Autodesk Fusion 360 part; units mm, degrees
(part 2 of 2)
sketch "Sketch5" plane through (0, 0, 0) normal (0, -1, 0) x (1, 0, 0)
  line L0 (114.0188, -15.2131) -> (113.0529, -22.5498)
  line L1 (113.0529, -22.5498) -> (82.3181, -18.5035)
  line L2 (82.3181, -18.5035) -> (83.284, -11.1668)
  line L3 (83.284, -11.1668) -> (114.0188, -15.2131)
  line L4 (138.2617, -49.6626) -> (131.6978, -53.0795)
  line L5 (131.6978, -53.0795) -> (117.3836, -25.5822)
  line L6 (117.3836, -25.5822) -> (123.9475, -22.1652)
  line L7 (123.9475, -22.1652) -> (138.2617, -49.6626)
  line L8 (56.4068, -68.2786) -> (77.3501, -91.1342)
  line L9 (77.3501, -91.1342) -> (71.8943, -96.1335)
  line L10 (71.8943, -96.1335) -> (50.951, -73.2779)
  line L11 (50.951, -73.2779) -> (56.4068, -68.2786)
  line L12 (123.9475, -89.2806) -> (117.3836, -85.8637)
  line L13 (117.3836, -85.8637) -> (131.6978, -58.3663)
  line L14 (131.6978, -58.3663) -> (138.2617, -61.7833)
  line L15 (138.2617, -61.7833) -> (123.9475, -89.2806)
  line L16 (83.284, -100.2791) -> (82.3181, -92.9424)
  line L17 (82.3181, -92.9424) -> (113.0529, -88.8961)
  line L18 (113.0529, -88.8961) -> (114.0188, -96.2328)
  line L19 (114.0188, -96.2328) -> (83.284, -100.2791)
  line L20 (71.8943, -15.3123) -> (77.3501, -20.3117)
  line L21 (77.3501, -20.3117) -> (56.4068, -43.1673)
  line L22 (56.4068, -43.1673) -> (50.951, -38.1679)
  line L23 (50.951, -38.1679) -> (71.8943, -15.3123)
  circle A0 centre (93.0518, -55.7229) radius 32
  line L24 (43.0518, -60.3246) -> (33.0518, -60.3246)
  line L25 (33.0518, -60.3246) -> (33.0518, -62.9729)
  arc A1 (33.0518, -62.9729) -> (35.0035, -66.9362) centre (38.0518, -62.9729) ccw
  spline S0 degree 5 poles (35.0035, -66.9362) (35.0877, -67.0016) (35.3696, -67.2106) (35.8903, -67.5453) (36.7154, -67.9795) (37.8844, -68.5138) (39.2185, -69.1644) (40.4642, -69.9451) (41.5622, -70.9096) (42.5171, -72.0738) (43.3656, -73.4352) (44.0003, -74.673) (44.4719, -75.6799) (44.7873, -76.3854) (44.9452, -76.7467) knots 0.055622 0.055622 0.055622 0.055622 0.055622 0.055622 0.1 0.2 0.3 0.4 0.5 0.6 0.7 0.8 0.9 1 1 1 1 1 1
  arc A2 (44.9452, -76.7467) -> (44.6036, -35.4987) centre (93.0518, -55.7229) ccw
  spline S1 degree 5 poles (35.0976, -44.439) (35.1635, -44.39) (35.4284, -44.1998) (35.929, -43.8843) (36.7276, -43.467) (37.8672, -42.9464) (39.2068, -42.2909) (40.468, -41.4976) (41.5888, -40.515) (42.5659, -39.3335) (43.3462, -38.0903) (43.9063, -37.0155) (44.2932, -36.1952) (44.5236, -35.6806) (44.6036, -35.4987) knots 0.065909 0.065909 0.065909 0.065909 0.065909 0.065909 0.1 0.2 0.3 0.4 0.5 0.6 0.7 0.8 0.9 0.95371 0.95371 0.95371 0.95371 0.95371 0.95371
  arc A3 (35.0976, -44.439) -> (33.0518, -48.4729) centre (38.0518, -48.4729) ccw
  line L26 (33.0518, -48.4729) -> (33.0518, -51.3246)
  line L27 (33.0518, -51.3246) -> (43.0518, -51.3246)
  line L28 (43.0518, -51.3246) -> (43.0518, -60.3246)
  circle A4 centre (93.0518, -55.7229) radius 32
  line L29 (56.4068, -43.1673) -> (77.3501, -20.3117)
  line L30 (50.951, -38.1679) -> (56.4068, -43.1673)
  line L31 (71.8943, -15.3123) -> (50.951, -38.1679)
  line L32 (77.3501, -20.3117) -> (71.8943, -15.3123)
  line L33 (113.0529, -88.8961) -> (82.3181, -92.9424)
  line L34 (114.0188, -96.2328) -> (113.0529, -88.8961)
  line L35 (83.284, -100.2791) -> (114.0188, -96.2328)
  line L36 (82.3181, -92.9424) -> (83.284, -100.2791)
  line L37 (131.6978, -58.3663) -> (117.3836, -85.8637)
  line L38 (138.2617, -61.7833) -> (131.6978, -58.3663)
  line L39 (123.9475, -89.2806) -> (138.2617, -61.7833)
  line L40 (117.3836, -85.8637) -> (123.9475, -89.2806)
  line L41 (71.8943, -96.1335) -> (77.3501, -91.1342)
  line L42 (50.951, -73.2779) -> (71.8943, -96.1335)
  line L43 (56.4068, -68.2786) -> (50.951, -73.2779)
  line L44 (77.3501, -91.1342) -> (56.4068, -68.2786)
  line L45 (117.3836, -25.5822) -> (131.6978, -53.0795)
  line L46 (123.9475, -22.1652) -> (117.3836, -25.5822)
  line L47 (138.2617, -49.6626) -> (123.9475, -22.1652)
  line L48 (131.6978, -53.0795) -> (138.2617, -49.6626)
  line L49 (82.3181, -18.5035) -> (113.0529, -22.5498)
  line L50 (83.284, -11.1668) -> (82.3181, -18.5035)
  line L51 (114.0188, -15.2131) -> (83.284, -11.1668)
  line L52 (113.0529, -22.5498) -> (114.0188, -15.2131)
  line L53 (33.0518, -62.9729) -> (33.0518, -60.3246)
  arc A5 (33.0518, -62.9729) -> (35.0035, -66.9362) centre (38.0518, -62.9729) ccw
  spline S2 degree 5 poles (44.9452, -76.7467) (44.7873, -76.3854) (44.4719, -75.6799) (44.0003, -74.673) (43.3656, -73.4352) (42.5171, -72.0738) (41.5622, -70.9096) (40.4642, -69.9451) (39.2185, -69.1644) (37.8844, -68.5138) (36.7154, -67.9795) (35.8903, -67.5453) (35.3696, -67.2106) (35.0877, -67.0016) (35.0035, -66.9362) knots -1 -1 -1 -1 -1 -1 -0.9 -0.8 -0.7 -0.6 -0.5 -0.4 -0.3 -0.2 -0.1 -0.055622 -0.055622 -0.055622 -0.055622 -0.055622 -0.055622
  arc A6 (44.9452, -76.7467) -> (44.6036, -35.4987) centre (93.0518, -55.7229) ccw
  spline S3 degree 5 poles (35.0976, -44.439) (35.1635, -44.39) (35.4284, -44.1998) (35.929, -43.8843) (36.7276, -43.467) (37.8672, -42.9464) (39.2068, -42.2909) (40.468, -41.4976) (41.5888, -40.515) (42.5659, -39.3335) (43.3462, -38.0903) (43.9063, -37.0155) (44.2932, -36.1952) (44.5236, -35.6806) (44.6036, -35.4987) knots 0.065909 0.065909 0.065909 0.065909 0.065909 0.065909 0.1 0.2 0.3 0.4 0.5 0.6 0.7 0.8 0.9 0.95371 0.95371 0.95371 0.95371 0.95371 0.95371
  arc A7 (35.0976, -44.439) -> (33.0518, -48.4729) centre (38.0518, -48.4729) ccw
  line L54 (33.0518, -51.3246) -> (33.0518, -48.4729)
  line L55 (43.0518, -51.3246) -> (33.0518, -51.3246)
  line L56 (43.0518, -60.3246) -> (43.0518, -51.3246)
  line L57 (33.0518, -60.3246) -> (43.0518, -60.3246)
  arc A8 (107.5518, -60.7229) -> (108.5518, -59.7229) centre (107.5518, -59.7229) ccw
  line L58 (105.5518, -60.7229) -> (107.5518, -60.7229)
  arc A9 (105.5518, -60.7229) -> (102.5518, -63.7229) centre (105.5518, -63.7229) ccw
  line L59 (108.5518, -63.7229) -> (102.5518, -63.7229)
  line L60 (108.5518, -66.7229) -> (108.5518, -63.7229)
  line L61 (103.5518, -66.7229) -> (108.5518, -66.7229)
  line L62 (103.5518, -69.7229) -> (103.5518, -66.7229)
  line L63 (108.5518, -69.7229) -> (103.5518, -69.7229)
  line L64 (108.5518, -72.7229) -> (108.5518, -69.7229)
  line L65 (93.5518, -72.7229) -> (108.5518, -72.7229)
  spline S4 degree 2 poles (103.5518, -77.7229) (93.5518, -77.7229) (93.5518, -72.7229) knots -1 -1 -1 0 0 0
  spline S5 degree 2 poles (113.5518, -72.7229) (113.5518, -77.7229) (103.5518, -77.7229) knots 0 0 0 1 1 1
  line L66 (113.5518, -60.7229) -> (113.5518, -72.7229)
  line L67 (113.5518, -44.7229) -> (113.5518, -60.7229)
  arc A10 (113.5518, -44.7229) -> (109.5518, -40.7229) centre (109.5518, -44.7229) ccw
  arc A11 (109.5518, -40.7229) -> (108.5518, -41.7229) centre (109.5518, -41.7229) ccw
  line L68 (108.5518, -59.7229) -> (108.5518, -41.7229)
  arc A12 (99.5518, -49.7229) -> (98.5518, -50.7229) centre (99.5518, -50.7229) ccw
  line L69 (101.5518, -49.7229) -> (99.5518, -49.7229)
  arc A13 (101.5518, -49.7229) -> (104.5518, -46.7229) centre (101.5518, -46.7229) ccw
  line L70 (98.5518, -46.7229) -> (104.5518, -46.7229)
  line L71 (98.5518, -43.7229) -> (98.5518, -46.7229)
  line L72 (103.5518, -43.7229) -> (98.5518, -43.7229)
  line L73 (103.5518, -40.7229) -> (103.5518, -43.7229)
  line L74 (98.5518, -40.7229) -> (103.5518, -40.7229)
  line L75 (98.5518, -37.7229) -> (98.5518, -40.7229)
  line L76 (113.5518, -37.7229) -> (98.5518, -37.7229)
  spline S6 degree 2 poles (103.5518, -32.7229) (113.5518, -32.7229) (113.5518, -37.7229) knots -1 -1 -1 0 0 0
  spline S7 degree 2 poles (93.5518, -37.7229) (93.5518, -32.7229) (103.5518, -32.7229) knots 0 0 0 1 1 1
  line L77 (93.5518, -49.7229) -> (93.5518, -37.7229)
  line L78 (93.5518, -65.7229) -> (93.5518, -49.7229)
  arc A14 (93.5518, -65.7229) -> (97.5518, -69.7229) centre (97.5518, -65.7229) ccw
  arc A15 (97.5518, -69.7229) -> (98.5518, -68.7229) centre (97.5518, -68.7229) ccw
  line L79 (98.5518, -50.7229) -> (98.5518, -68.7229)
  arc A16 (85.0518, -60.7229) -> (86.0518, -59.7229) centre (85.0518, -59.7229) ccw
  line L80 (83.0518, -60.7229) -> (85.0518, -60.7229)
  arc A17 (83.0518, -60.7229) -> (80.0518, -63.7229) centre (83.0518, -63.7229) ccw
  line L81 (86.0518, -63.7229) -> (80.0518, -63.7229)
  line L82 (86.0518, -66.7229) -> (86.0518, -63.7229)
  line L83 (81.0518, -66.7229) -> (86.0518, -66.7229)
  line L84 (81.0518, -69.7229) -> (81.0518, -66.7229)
  line L85 (86.0518, -69.7229) -> (81.0518, -69.7229)
  line L86 (86.0518, -72.7229) -> (86.0518, -69.7229)
  line L87 (71.0518, -72.7229) -> (86.0518, -72.7229)
  spline S8 degree 2 poles (81.0518, -77.7229) (71.0518, -77.7229) (71.0518, -72.7229) knots -1 -1 -1 0 0 0
  spline S9 degree 2 poles (91.0518, -72.7229) (91.0518, -77.7229) (81.0518, -77.7229) knots 0 0 0 1 1 1
  line L88 (91.0518, -60.7229) -> (91.0518, -72.7229)
  line L89 (91.0518, -44.7229) -> (91.0518, -60.7229)
  arc A18 (91.0518, -44.7229) -> (87.0518, -40.7229) centre (87.0518, -44.7229) ccw
  arc A19 (87.0518, -40.7229) -> (86.0518, -41.7229) centre (87.0518, -41.7229) ccw
  line L90 (86.0518, -59.7229) -> (86.0518, -41.7229)
  arc A20 (77.0518, -49.7229) -> (76.0518, -50.7229) centre (77.0518, -50.7229) ccw
  line L91 (79.0518, -49.7229) -> (77.0518, -49.7229)
  arc A21 (79.0518, -49.7229) -> (82.0518, -46.7229) centre (79.0518, -46.7229) ccw
  line L92 (76.0518, -46.7229) -> (82.0518, -46.7229)
  line L93 (76.0518, -43.7229) -> (76.0518, -46.7229)
  line L94 (81.0518, -43.7229) -> (76.0518, -43.7229)
  line L95 (81.0518, -40.7229) -> (81.0518, -43.7229)
  line L96 (76.0518, -40.7229) -> (81.0518, -40.7229)
  line L97 (76.0518, -37.7229) -> (76.0518, -40.7229)
  line L98 (91.0518, -37.7229) -> (76.0518, -37.7229)
  spline S10 degree 2 poles (81.0518, -32.7229) (91.0518, -32.7229) (91.0518, -37.7229) knots -1 -1 -1 0 0 0
  spline S11 degree 2 poles (71.0518, -37.7229) (71.0518, -32.7229) (81.0518, -32.7229) knots 0 0 0 1 1 1
  line L99 (71.0518, -49.7229) -> (71.0518, -37.7229)
  line L100 (71.0518, -65.7229) -> (71.0518, -49.7229)
  arc A22 (71.0518, -65.7229) -> (75.0518, -69.7229) centre (75.0518, -65.7229) ccw
  arc A23 (75.0518, -69.7229) -> (76.0518, -68.7229) centre (75.0518, -68.7229) ccw
  line L101 (76.0518, -50.7229) -> (76.0518, -68.7229)
  circle A24 centre (0, -110) radius 32
  spline S12 degree 5 poles (48.1066, -88.9762) (48.2645, -89.3375) (48.5799, -90.043) (49.0515, -91.0499) (49.6862, -92.2877) (50.5348, -93.6491) (51.4896, -94.8133) (52.5876, -95.7778) (53.8333, -96.5585) (55.1674, -97.2091) (56.3365, -97.7434) (57.1616, -98.1776) (57.6822, -98.5123) (57.9641, -98.7213) (58.0483, -98.7867) knots -1 -1 -1 -1 -1 -1 -0.9 -0.8 -0.7 -0.6 -0.5 -0.4 -0.3 -0.2 -0.1 -0.055622 -0.055622 -0.055622 -0.055622 -0.055622 -0.055622
  arc A25 (48.1066, -88.9762) -> (48.4482, -130.2242) centre (0, -110) ccw
  spline S13 degree 5 poles (57.9542, -121.2839) (57.8883, -121.3329) (57.6234, -121.5231) (57.1228, -121.8387) (56.3243, -122.2559) (55.1846, -122.7765) (53.845, -123.4321) (52.5838, -124.2253) (51.463, -125.2079) (50.4859, -126.3894) (49.7057, -127.6326) (49.1456, -128.7074) (48.7586, -129.5278) (48.5283, -130.0423) (48.4482, -130.2242) knots 0.065909 0.065909 0.065909 0.065909 0.065909 0.065909 0.1 0.2 0.3 0.4 0.5 0.6 0.7 0.8 0.9 0.95371 0.95371 0.95371 0.95371 0.95371 0.95371
  arc A26 (57.9542, -121.2839) -> (60, -117.25) centre (55, -117.25) ccw
  line L102 (60, -102.75) -> (60, -117.25)
  arc A27 (60, -102.75) -> (58.0483, -98.7867) centre (55, -102.75) ccw
  arc A28 (16, -116) -> (17, -115) centre (16, -115) ccw
  line L103 (14, -116) -> (16, -116)
  arc A29 (14, -116) -> (11, -119) centre (14, -119) ccw
  line L104 (17, -119) -> (11, -119)
  line L105 (17, -122) -> (17, -119)
  line L106 (12, -122) -> (17, -122)
  line L107 (12, -125) -> (12, -122)
  line L108 (17, -125) -> (12, -125)
  line L109 (17, -128) -> (17, -125)
  line L110 (2, -128) -> (17, -128)
  spline S14 degree 2 poles (12, -133) (2, -133) (2, -128) knots -1 -1 -1 0 0 0
  spline S15 degree 2 poles (22, -128) (22, -133) (12, -133) knots 0 0 0 1 1 1
  line L111 (22, -116) -> (22, -128)
  line L112 (22, -100) -> (22, -116)
  arc A30 (22, -100) -> (18, -96) centre (18, -100) ccw
  arc A31 (18, -96) -> (17, -97) centre (18, -97) ccw
  line L113 (17, -115) -> (17, -97)
  arc A32 (8, -105) -> (7, -106) centre (8, -106) ccw
  line L114 (10, -105) -> (8, -105)
  arc A33 (10, -105) -> (13, -102) centre (10, -102) ccw
  line L115 (7, -102) -> (13, -102)
  line L116 (7, -99) -> (7, -102)
  line L117 (12, -99) -> (7, -99)
  line L118 (12, -96) -> (12, -99)
  line L119 (7, -96) -> (12, -96)
  line L120 (7, -93) -> (7, -96)
  line L121 (22, -93) -> (7, -93)
  spline S16 degree 2 poles (12, -88) (22, -88) (22, -93) knots -1 -1 -1 0 0 0
  spline S17 degree 2 poles (2, -93) (2, -88) (12, -88) knots 0 0 0 1 1 1
  line L122 (2, -105) -> (2, -93)
  line L123 (2, -121) -> (2, -105)
  arc A34 (2, -121) -> (6, -125) centre (6, -121) ccw
  arc A35 (6, -125) -> (7, -124) centre (6, -124) ccw
  line L124 (7, -106) -> (7, -124)
  arc A36 (-14.5, -105) -> (-15.5, -106) centre (-14.5, -106) ccw
  line L125 (-12.5, -105) -> (-14.5, -105)
  arc A37 (-12.5, -105) -> (-9.5, -102) centre (-12.5, -102) ccw
  line L126 (-15.5, -102) -> (-9.5, -102)
  line L127 (-15.5, -99) -> (-15.5, -102)
  line L128 (-10.5, -99) -> (-15.5, -99)
  line L129 (-10.5, -96) -> (-10.5, -99)
  line L130 (-15.5, -96) -> (-10.5, -96)
  line L131 (-15.5, -93) -> (-15.5, -96)
  line L132 (-0.5, -93) -> (-15.5, -93)
  spline S18 degree 2 poles (-10.5, -88) (-0.5, -88) (-0.5, -93) knots -1 -1 -1 0 0 0
  spline S19 degree 2 poles (-20.5, -93) (-20.5, -88) (-10.5, -88) knots 0 0 0 1 1 1
  line L133 (-20.5, -105) -> (-20.5, -93)
  line L134 (-20.5, -121) -> (-20.5, -105)
  arc A38 (-20.5, -121) -> (-16.5, -125) centre (-16.5, -121) ccw
  arc A39 (-16.5, -125) -> (-15.5, -124) centre (-16.5, -124) ccw
  line L135 (-15.5, -106) -> (-15.5, -124)
  arc A40 (-6.5, -116) -> (-5.5, -115) centre (-6.5, -115) ccw
  line L136 (-8.5, -116) -> (-6.5, -116)
  arc A41 (-8.5, -116) -> (-11.5, -119) centre (-8.5, -119) ccw
  line L137 (-5.5, -119) -> (-11.5, -119)
  line L138 (-5.5, -122) -> (-5.5, -119)
  line L139 (-10.5, -122) -> (-5.5, -122)
  line L140 (-10.5, -125) -> (-10.5, -122)
  line L141 (-5.5, -125) -> (-10.5, -125)
  line L142 (-5.5, -128) -> (-5.5, -125)
  line L143 (-20.5, -128) -> (-5.5, -128)
  spline S20 degree 2 poles (-10.5, -133) (-20.5, -133) (-20.5, -128) knots -1 -1 -1 0 0 0
  spline S21 degree 2 poles (-0.5, -128) (-0.5, -133) (-10.5, -133) knots 0 0 0 1 1 1
  line L144 (-0.5, -116) -> (-0.5, -128)
  line L145 (-0.5, -100) -> (-0.5, -116)
  arc A42 (-0.5, -100) -> (-4.5, -96) centre (-4.5, -100) ccw
  arc A43 (-4.5, -96) -> (-5.5, -97) centre (-4.5, -97) ccw
  line L146 (-5.5, -115) -> (-5.5, -97)
  circle A44 centre (0, 0) radius 32
  line L147 (-1.5, 52.4786) -> (-1.5, 47.5)
  arc A45 (-1.5, 52.4786) -> (-44.6978, 27.5383) centre (0, 0) ccw
  line L148 (-40.3862, 25.049) -> (-44.6978, 27.5383)
  line L149 (-41.8862, 22.451) -> (-40.3862, 25.049)
  line L150 (-46.1978, 24.9402) -> (-41.8862, 22.451)
  arc A46 (-46.1978, 24.9402) -> (-46.1978, -24.9402) centre (0, 0) ccw
  line L151 (-41.8862, -22.451) -> (-46.1978, -24.9402)
  line L152 (-40.3862, -25.049) -> (-41.8862, -22.451)
  line L153 (-44.6978, -27.5383) -> (-40.3862, -25.049)
  arc A47 (-44.6978, -27.5383) -> (-1.5, -52.4786) centre (0, 0) ccw
  line L154 (-1.5, -47.5) -> (-1.5, -52.4786)
  line L155 (1.5, -47.5) -> (-1.5, -47.5)
  line L156 (1.5, -52.4786) -> (1.5, -47.5)
  arc A48 (1.5, -52.4786) -> (44.6978, -27.5383) centre (0, 0) ccw
  line L157 (40.3862, -25.049) -> (44.6978, -27.5383)
  line L158 (41.8862, -22.451) -> (40.3862, -25.049)
  line L159 (46.1978, -24.9402) -> (41.8862, -22.451)
  arc A49 (46.1978, -24.9402) -> (48.1066, -21.0238) centre (0, 0) ccw
  spline S22 degree 5 poles (48.4482, -20.2242) (48.3793, -20.381) (48.3106, -20.5394) (48.2423, -20.6993) (48.1743, -20.8608) (48.1066, -21.0238) knots 0.95371 0.95371 0.95371 0.95371 0.95371 0.95371 1 1 1 1 1 1
  spline S23 degree 5 poles (57.9542, -11.2839) (57.8883, -11.3329) (57.6234, -11.5231) (57.1228, -11.8387) (56.3243, -12.2559) (55.1846, -12.7765) (53.845, -13.4321) (52.5838, -14.2253) (51.463, -15.2079) (50.4859, -16.3894) (49.7057, -17.6326) (49.1456, -18.7074) (48.7586, -19.5278) (48.5283, -20.0423) (48.4482, -20.2242) knots 0.065909 0.065909 0.065909 0.065909 0.065909 0.065909 0.1 0.2 0.3 0.4 0.5 0.6 0.7 0.8 0.9 0.95371 0.95371 0.95371 0.95371 0.95371 0.95371
  spline S24 degree 5 poles (58.5355, -10.7855) (58.4307, -10.8904) (58.3201, -10.9926) (58.2037, -11.0922) (58.0816, -11.1892) (57.9542, -11.2839) knots 0 0 0 0 0 0 0.065909 0.065909 0.065909 0.065909 0.065909 0.065909
  arc A50 (58.5355, -10.7855) -> (60, -7.25) centre (55, -7.25) ccw
  line L160 (60, -4.3983) -> (60, -7.25)
  line L161 (57, -4.3983) -> (60, -4.3983)
  line L162 (57, -9.25) -> (57, -4.3983)
  line L163 (34, -9.25) -> (57, -9.25)
  line L164 (34, 9.25) -> (34, -9.25)
  line L165 (36.8706, 9.25) -> (34, 9.25)
  arc A51 (36.8706, 9.25) -> (36.5525, 10.4364) centre (0, 0) ccw
  line L166 (13.5824, 35.5038) -> (36.5525, 10.4364)
  arc A52 (13.5824, 35.5038) -> (12.4167, 35.9281) centre (0, 0) ccw
  line L167 (-21.2925, 31.4902) -> (12.4167, 35.9281)
  arc A53 (-21.2925, 31.4902) -> (-22.3086, 30.7786) centre (0, 0) ccw
  line L168 (-38.0081, 0.6203) -> (-22.3086, 30.7786)
  arc A54 (-38.0081, 0.6203) -> (-38.0081, -0.6203) centre (0, 0) ccw
  line L169 (-22.3086, -30.7786) -> (-38.0081, -0.6203)
  arc A55 (-22.3086, -30.7786) -> (-21.2925, -31.4902) centre (0, 0) ccw
  line L170 (12.4167, -35.9281) -> (-21.2925, -31.4902)
  arc A56 (12.4167, -35.9281) -> (13.5824, -35.5038) centre (0, 0) ccw
  line L171 (34.8906, -12.25) -> (13.5824, -35.5038)
  line L172 (38.5317, -12.25) -> (34.8906, -12.25)
  line L173 (44.2201, -17.4625) -> (38.5317, -12.25)
  line L174 (21.2501, -42.5299) -> (44.2201, -17.4625)
  arc A57 (11.0592, -46.2391) -> (21.2501, -42.5299) centre (0, 0) ccw
  line L175 (-22.6499, -41.8012) -> (11.0592, -46.2391)
  arc A58 (-31.5336, -35.5808) -> (-22.6499, -41.8012) centre (0, 0) ccw
  line L176 (-47.233, -5.4225) -> (-31.5336, -35.5808)
  arc A59 (-47.233, 5.4225) -> (-47.233, -5.4225) centre (0, 0) ccw
  line L177 (-31.5336, 35.5808) -> (-47.233, 5.4225)
  arc A60 (-22.6499, 41.8012) -> (-31.5336, 35.5808) centre (0, 0) ccw
  line L178 (11.0592, 46.2391) -> (-22.6499, 41.8012)
  arc A61 (21.2501, 42.5299) -> (11.0592, 46.2391) centre (0, 0) ccw
  line L179 (44.2201, 17.4625) -> (21.2501, 42.5299)
  spline S25 degree 5 poles (51.3871, 10.7526) (51.0937, 10.9213) (50.1955, 11.4779) (48.7982, 12.541) (47.0834, 14.2002) (45.7147, 15.761) (44.8358, 16.7778) (44.4003, 17.2659) (44.2201, 17.4625) knots 0.306371 0.306371 0.306371 0.306371 0.306371 0.306371 0.4 0.6 0.8 1 1 1 1 1 1
  spline S26 degree 5 poles (57, 9.25) (56.1534, 9.25) (54.916, 9.3573) (53.7693, 9.6287) (52.7064, 10.0415) (51.7204, 10.561) (51.3871, 10.7526) knots 0 0 0 0 0 0 0.2 0.306371 0.306371 0.306371 0.306371 0.306371 0.306371
  line L180 (57, 4.6017) -> (57, 9.25)
  line L181 (60, 4.6017) -> (57, 4.6017)
  line L182 (60, 7.25) -> (60, 4.6017)
  arc A62 (60, 7.25) -> (58.5355, 10.7855) centre (55, 7.25) ccw
  spline S27 degree 5 poles (58.0483, 11.2133) (58.1538, 11.1314) (58.2553, 11.0477) (58.3529, 10.9622) (58.4463, 10.8748) (58.5355, 10.7855) knots -0.055622 -0.055622 -0.055622 -0.055622 -0.055622 -0.055622 0 0 0 0 0 0
  spline S28 degree 5 poles (48.1066, 21.0238) (48.2645, 20.6625) (48.5799, 19.957) (49.0515, 18.9501) (49.6862, 17.7123) (50.5348, 16.3509) (51.4896, 15.1867) (52.5876, 14.2222) (53.8333, 13.4415) (55.1674, 12.7909) (56.3365, 12.2566) (57.1616, 11.8224) (57.6822, 11.4877) (57.9641, 11.2787) (58.0483, 11.2133) knots -1 -1 -1 -1 -1 -1 -0.9 -0.8 -0.7 -0.6 -0.5 -0.4 -0.3 -0.2 -0.1 -0.055622 -0.055622 -0.055622 -0.055622 -0.055622 -0.055622
  arc A63 (48.1066, 21.0238) -> (46.1978, 24.9402) centre (0, 0) ccw
  line L183 (41.8862, 22.451) -> (46.1978, 24.9402)
  line L184 (40.3862, 25.049) -> (41.8862, 22.451)
  line L185 (44.6978, 27.5383) -> (40.3862, 25.049)
  arc A64 (44.6978, 27.5383) -> (1.5, 52.4786) centre (0, 0) ccw
  line L186 (1.5, 47.5) -> (1.5, 52.4786)
  line L187 (-1.5, 47.5) -> (1.5, 47.5)
  arc A65 (16, -6) -> (17, -5) centre (16, -5) ccw
  line L188 (14, -6) -> (16, -6)
  arc A66 (14, -6) -> (11, -9) centre (14, -9) ccw
  line L189 (17, -9) -> (11, -9)
  line L190 (17, -12) -> (17, -9)
  line L191 (12, -12) -> (17, -12)
  line L192 (12, -15) -> (12, -12)
  line L193 (17, -15) -> (12, -15)
  line L194 (17, -18) -> (17, -15)
  line L195 (2, -18) -> (17, -18)
  spline S29 degree 2 poles (12, -23) (2, -23) (2, -18) knots -1 -1 -1 0 0 0
  spline S30 degree 2 poles (22, -18) (22, -23) (12, -23) knots 0 0 0 1 1 1
  line L196 (22, -6) -> (22, -18)
  line L197 (22, 10) -> (22, -6)
  arc A67 (22, 10) -> (18, 14) centre (18, 10) ccw
  arc A68 (18, 14) -> (17, 13) centre (18, 13) ccw
  line L198 (17, -5) -> (17, 13)
  arc A69 (8, 5) -> (7, 4) centre (8, 4) ccw
  line L199 (10, 5) -> (8, 5)
  arc A70 (10, 5) -> (13, 8) centre (10, 8) ccw
  line L200 (7, 8) -> (13, 8)
  line L201 (7, 11) -> (7, 8)
  line L202 (12, 11) -> (7, 11)
  line L203 (12, 14) -> (12, 11)
  line L204 (7, 14) -> (12, 14)
  line L205 (7, 17) -> (7, 14)
  line L206 (22, 17) -> (7, 17)
  spline S31 degree 2 poles (12, 22) (22, 22) (22, 17) knots -1 -1 -1 0 0 0
  spline S32 degree 2 poles (2, 17) (2, 22) (12, 22) knots 0 0 0 1 1 1
  line L207 (2, 5) -> (2, 17)
  line L208 (2, -11) -> (2, 5)
  arc A71 (2, -11) -> (6, -15) centre (6, -11) ccw
  arc A72 (6, -15) -> (7, -14) centre (6, -14) ccw
  line L209 (7, 4) -> (7, -14)
  arc A73 (-6.5, -6) -> (-5.5, -5) centre (-6.5, -5) ccw
  line L210 (-8.5, -6) -> (-6.5, -6)
  arc A74 (-8.5, -6) -> (-11.5, -9) centre (-8.5, -9) ccw
  line L211 (-5.5, -9) -> (-11.5, -9)
  line L212 (-5.5, -12) -> (-5.5, -9)
  line L213 (-10.5, -12) -> (-5.5, -12)
  line L214 (-10.5, -15) -> (-10.5, -12)
  line L215 (-5.5, -15) -> (-10.5, -15)
  line L216 (-5.5, -18) -> (-5.5, -15)
  line L217 (-20.5, -18) -> (-5.5, -18)
  spline S33 degree 2 poles (-10.5, -23) (-20.5, -23) (-20.5, -18) knots -1 -1 -1 0 0 0
  spline S34 degree 2 poles (-0.5, -18) (-0.5, -23) (-10.5, -23) knots 0 0 0 1 1 1
  line L218 (-0.5, -6) -> (-0.5, -18)
  line L219 (-0.5, 10) -> (-0.5, -6)
  arc A75 (-0.5, 10) -> (-4.5, 14) centre (-4.5, 10) ccw
  arc A76 (-4.5, 14) -> (-5.5, 13) centre (-4.5, 13) ccw
  line L220 (-5.5, -5) -> (-5.5, 13)
  arc A77 (-14.5, 5) -> (-15.5, 4) centre (-14.5, 4) ccw
  line L221 (-12.5, 5) -> (-14.5, 5)
  arc A78 (-12.5, 5) -> (-9.5, 8) centre (-12.5, 8) ccw
  line L222 (-15.5, 8) -> (-9.5, 8)
  line L223 (-15.5, 11) -> (-15.5, 8)
  line L224 (-10.5, 11) -> (-15.5, 11)
  line L225 (-10.5, 14) -> (-10.5, 11)
  line L226 (-15.5, 14) -> (-10.5, 14)
  line L227 (-15.5, 17) -> (-15.5, 14)
  line L228 (-0.5, 17) -> (-15.5, 17)
  spline S35 degree 2 poles (-10.5, 22) (-0.5, 22) (-0.5, 17) knots -1 -1 -1 0 0 0
  spline S36 degree 2 poles (-20.5, 17) (-20.5, 22) (-10.5, 22) knots 0 0 0 1 1 1
  line L229 (-20.5, 5) -> (-20.5, 17)
  line L230 (-20.5, -11) -> (-20.5, 5)
  arc A79 (-20.5, -11) -> (-16.5, -15) centre (-16.5, -11) ccw
  arc A80 (-16.5, -15) -> (-15.5, -14) centre (-16.5, -14) ccw
  line L231 (-15.5, 4) -> (-15.5, -14)
copy_body "CopyPasteBodies5" [suppressed]
move_body "Move17" [suppressed]
move_body "Move18" [suppressed]
move_body "Move19" [suppressed]
move_body "Move20" [suppressed]
move_body "Move21" [suppressed]
move_body "Move22" [suppressed]
sketch "Sketch4" plane through (0, 6, 0) normal (0, 1, 0) x (-1, 0, 0)
  circle A0 centre (-300, 0) radius 32
  arc A1 (-358.0483, 11.2133) -> (-360, 7.25) centre (-355, 7.25) ccw
  line L0 (-360, 7.25) -> (-360, -7.25)
  arc A2 (-360, -7.25) -> (-357.9542, -11.2839) centre (-355, -7.25) ccw
  spline S0 degree 5 poles (-357.9542, -11.2839) (-357.8883, -11.3329) (-357.6234, -11.5231) (-357.1228, -11.8387) (-356.3243, -12.2559) (-355.1846, -12.7765) (-353.845, -13.4321) (-352.5838, -14.2253) (-351.463, -15.2079) (-350.4859, -16.3894) (-349.7057, -17.6326) (-349.1456, -18.7074) (-348.7586, -19.5278) (-348.5283, -20.0423) (-348.4482, -20.2242) knots 0.065909 0.065909 0.065909 0.065909 0.065909 0.065909 0.1 0.2 0.3 0.4 0.5 0.6 0.7 0.8 0.9 0.95371 0.95371 0.95371 0.95371 0.95371 0.95371
  arc A3 (-348.4482, -20.2242) -> (-348.1066, 21.0238) centre (-300, 0) ccw
  spline S1 degree 5 poles (-348.1066, 21.0238) (-348.2645, 20.6625) (-348.5799, 19.957) (-349.0515, 18.9501) (-349.6862, 17.7123) (-350.5348, 16.3509) (-351.4896, 15.1867) (-352.5876, 14.2222) (-353.8333, 13.4415) (-355.1674, 12.7909) (-356.3365, 12.2566) (-357.1616, 11.8224) (-357.6822, 11.4877) (-357.9641, 11.2787) (-358.0483, 11.2133) knots -1 -1 -1 -1 -1 -1 -0.9 -0.8 -0.7 -0.6 -0.5 -0.4 -0.3 -0.2 -0.1 -0.055622 -0.055622 -0.055622 -0.055622 -0.055622 -0.055622
  line L1 (-300, -32) -> (-300, 32)
  line L2 (-268, 0) -> (-332, 0)
  constraint coincident A0 L1.start
  constraint coincident A0 L1.end
  constraint vertical L1
  constraint coincident A0 L2.start
  constraint coincident A0 L2.end
  constraint perpendicular L1 L2
pattern_circular "C-Pattern1" [suppressed]
move_body "Move23" [suppressed]
move_body "Move24" [suppressed]
equation "d8 = ( 18.5 / 2 ) * 1 mm"
